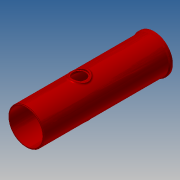
# Autodesk Inventor part: A1-19027-400-07 HCWI liner - trunk
Saved by Autodesk Inventor 2017.3 (Build 213257000, 257)
## iProperties
Created: 2019-08-16
Part Number: A1-19027-400-07 HCWI liner - trunk
Material: Iron, HCWI
Document SubType Name: Modeling
Designer: GVD
Density: 7.33517 g/cm^3
Appearance: Iron Gray(1)
Mass: 1.55202e+06 g
Surface Area: 133734 cm^2
Volume: 211585 cm^3
Description: 28 1/2" ID x 1 1/4" WALL x 110" HCWI LINER w/ DRAINS, ASTM A532 CLASS III TYPE A, PF# 470299
Author: GVD
Autodesk Inventor part; units mm, degrees
ref_plane "YZ Plane" through (0, 0, 0) normal (1, 0, 0) x (0, 1, 0)
ref_plane "XY Plane" through (0, 0, 0) normal (0, 0, 1) x (1, 0, 0)
sketch "Sketch1" plane through (0, 0, 0) normal (0, 0, 1) x (1, 0, 0)
  circle A0 centre (0, 0) radius 361.95
  circle A1 centre (0, 0) radius 393.7
  dimension "d0" = 723.9
  dimension "d1" = 787.4
  constraints: 2 centre point, 2 coincident
  measures "d0" diameter of A0
  measures "d1" diameter of A1
extrude "Extrusion1" add sketch "Sketch1" along normal blind 2794
sketch "Sketch2" plane through (0, 0, 0) normal (0, 0, -1) x (-1, 0, 0)
  circle A0 centre (0, 0) radius 393.7 projected
  circle A1 centre (0, 0) radius 415.925
  dimension "d4" = 831.85
  constraints: 1 centre point, 1 coincident
  measures "d4" diameter of A1
extrude "Extrusion2" add sketch "Sketch2" against normal blind 50.8
sketch "Sketch3" plane through (0, 0, 0) normal (0, 0, -1) x (-1, 0, 0)
  circle A0 centre (0, 0) radius 415.925 projected
  circle A1 centre (0, 0) radius 412.496
  dimension "d7" = 824.992
  constraints: 1 centre point, 1 coincident
  measures "d7" diameter of A1
extrude "Extrusion3" cut sketch "Sketch3" against normal blind 25.4
chamfer "Chamfer1" distance 22.225 angle 45 1 edges at (-393.7, 0, 50.8)
sketch "Sketch4" plane through (0, 0, 2794) normal (0, 0, 1) x (1, 0, 0)
  circle A0 centre (0, 0) radius 393.7 projected
  circle A1 centre (0, 0) radius 380.746
  dimension "d13" = 761.492
  constraints: 1 centre point, 1 coincident
  measures "d13" diameter of A1
extrude "Extrusion4" cut sketch "Sketch4" against normal blind 12.7
chamfer "Chamfer2" distance 0.7937 angle 45 1 edges at (-380.746, 0, 2794)
fillet "Fillet1" radius 0.7937 2 edges at (-380.746, 0, 2781.3) (412.496, 0, 25.4)
sketch "Sketch5" plane through (0, 0, 0) normal (0, 1, 0) x (-1, 0, 0)
  circle A0 centre (0, 440) radius 33
  circle A1 centre (0, 1633) radius 141.5
  point P0 (0, 0)
  dimension "d20" = 66
  dimension "d21" = 440
  dimension "d22" = 283
  dimension "d23" = 1193
  constraints: 2 centre point, 2 vertical alignment
  measures "d20" diameter of A0
  measures "d21" distance of point (0, 0) A0.centre
  measures "d22" diameter of A1
  measures "d23" distance of A0.centre A1.centre
extrude "Extrusion5" cut sketch "Sketch5" along normal through all both and the other way through all contours A1
ref_plane "Work Plane3" through (0, 469.9, 0) normal (0, 1, 0) x (-1, 0, 0)
ref_plane "Work Plane2" through (0, 393.7, 0) normal (0, 1, 0) x (-1, 0, 0)
sketch "Sketch7" plane through (0, 393.7, 0) normal (0, 1, 0) x (-1, 0, 0)
  circle A0 centre (0, 1633) radius 141.5 projected
  circle A1 centre (0, 1633) radius 192.3
  circle A2 centre (0, 1633) radius 161.925
  point P0 (0, 0)
  dimension "d39" = 384.6
  dimension "d42" = 323.85
  constraints: 2 centre point, 2 coincident
  measures "d39" diameter of A1
  measures "d42" diameter of A2
extrude "Extrusion9" add sketch "Sketch7" against normal up to surface contours A1 | A2 round surface about axis through (0, 0, 0) along (0, 0, 1) radius 393.7 far side no
extrude "Extrusion11" add sketch "Sketch7" along normal up to surface (76.2 mm away) contours A1
sketch "Sketch9" plane through (0, 469.9, 1633) normal (0, 1, 0) x (1, 0, 0)
  circle A0 centre (0, 0) radius 161.925 projected
  circle A1 centre (0, 0) radius 192.3 projected
  point P0 (0, 1633)
sketch "Sketch8" plane through (0, 0, 0) normal (0, 0, 1) x (1, 0, 0)
  circle A0 centre (0, 0) radius 415.925
  dimension "d43" = 831.85
  constraints: 1 centre point, 1 coincident
  measures "d43" diameter of A0
surface extrude "ExtrusionSrf1" sketch "Sketch8" along normal blind 2794 shown no curves A0
extrude "Extrusion12" cut sketch "Sketch9" against normal up to surface round surface about axis through (0, 0, 0) along (0, 0, 1) radius 415.925 far side no
extrude "Extrusion13" cut sketch "Sketch7" against normal blind 12.7 contours A2
fillet "Fillet3" radius 50.8 3 edges at (-146.3123, 365.5029, 1508.2122) (-146.3126, 365.5028, 1757.7875) (192.3, 343.541, 1632.9991)
fillet "Fillet5" radius 0.7937 1 edges at (161.925, 381, 1633)
pattern_circular "Circular Pattern2" count 2 over 360 about axis through (0, 0, -10) along (0, 0, 1) of "Extrusion9", "Fillet3", "Extrusion11", "Extrusion12", "Fillet5", "Extrusion13"
equation "\"d10\" = -0.5 * d1 + 0.5 * d4"
equation "\"d44\" = d2"
equation "\"d2\" = 2794"
body "Solid1"
body "Srf1"
